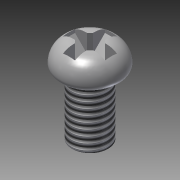
# Autodesk Inventor part: screw_M3_5
Saved by Autodesk Inventor 2013 (Build 170138000, 138)
## iProperties
Shininess: 20.0
Created: 2011-05-14
Part Number: screw_M3_5
Document SubType Name: Modeling
Designer: Noa Izumi
Material: Default
Density: 1 g/cm^3
Density: 0.0
Volumn: 0.0
Area: 0.0
PropertySet Name: Model Information
Control State: 0
Master: False
Checked Out: False
Author: Noa Izumi
Autodesk Inventor part; units mm, degrees
ref_plane "YZ Plane" through (0, 0, 0) normal (1, 0, 0) x (0, 1, 0)
ref_plane "XZ Plane" through (0, 0, 0) normal (0, 1, 0) x (-1, 0, 0)
ref_plane "XY Plane" through (0, 0, 0) normal (0, 0, 1) x (1, 0, 0)
sketch "Sketch1" plane through (0, 0, 0) normal (0, 0, 1) x (1, 0, 0)
  circle A0 centre (0, 0) radius 2.5
  dimension "d0" = 5
  constraints: 1 centre point
  measures "d0" diameter of A0
extrude "Extrusion1" add sketch "Sketch1" along normal blind 2
fillet "Fillet1" radius 0.5 1 edges at (-2.5, 0, 0)
fillet "Fillet2" radius 1.5 1 edges at (-2.5, 0, 2)
sketch "Sketch2" plane through (0, 0, 2) normal (0, 0, 1) x (1, 0, 0)
  circle A0 centre (0, 0) radius 1 projected
  line L0 (1.75, 0.5) -> (1.75, -0.5)
  line L1 (-1.75, -0.5) -> (-1.75, 0.5)
  line L2 (-0.5, 1.75) -> (0.5, 1.75)
  line L3 (0.5, -1.75) -> (-0.5, -1.75)
  line L4 (-0.5, -1.75) -> (-0.5, -0.5)
  line L5 (-0.5, 0.5) -> (-0.5, 1.75)
  line L6 (-1.75, 0.5) -> (-0.5, 0.5)
  line L7 (0.5, 0.5) -> (1.75, 0.5)
  line L8 (0.5, 1.75) -> (0.5, 0.5)
  line L9 (0.5, -0.5) -> (0.5, -1.75)
  line L10 (1.75, -0.5) -> (0.5, -0.5)
  line L11 (-0.5, -0.5) -> (-1.75, -0.5)
  dimension "d5" = 1
  dimension "d6" = 3.5
  dimension "d7" = 1.75
  dimension "d9" = 1
  dimension "d10" = 3.5
  dimension "d11" = 1.75
  constraints: 24 end point, 10 parallel, 4 perpendicular, 3 horizontal
  measures "d5" distance of L1.start L1.end
  measures "d6" distance of L1.end L0.start
  measures "d7" distance from line of L1 A0.centre
  measures "d9" distance of L2.start L2.end
  measures "d10" distance of L2.end L3.start
  measures "d11" distance from line of A0.centre L2
extrude "Extrusion2" cut sketch "Sketch2" against normal blind 1.5 contours A0 L10 L9 L4 L11 L6 L5 L8 L7 | A0 L7 L0 L10 | A0 L5 L2 L8 | L9 L3 L4 A0 | A0 L11 L1 L6
chamfer "Chamfer1" distance 1 angle 45 4 edges at (-1.75, 0, 0.5) (0, 1.75, 0.5) (1.75, 0, 0.5) (0, -1.75, 0.5)
chamfer "Chamfer2" distance 0.25 angle 45 4 edges at (-0.5, 0.5, 1.25) (-0.5, -0.5, 1.25) (0.5, 0.5, 1.25) (0.5, -0.5, 1.25)
sketch "Sketch3" plane through (0, 0, 0) normal (0, 0, -1) x (-1, 0, 0)
  circle A0 centre (0, 0) radius 2 projected
  circle A1 centre (0, 0) radius 1.5
  dimension "d19" = 3
  constraints: 1 centre point, 1 coincident
  measures "d19" diameter of A1
extrude "Extrusion3" add sketch "Sketch3" along normal blind 5 contours A1
thread "Thread1" size "M3x0.5" class "6g" standard "ANSI Metric M Profile" full length
